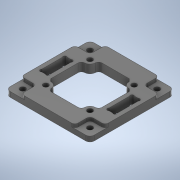
# Autodesk Inventor part: Camera_root_frame_e-CAM50_CUNX
Saved by Autodesk Inventor 2020.4 (Build 244396000, 396)
## iProperties
Part Number: Camera_root_frame_e-CAM50_CUNX
Material: アセタール樹脂、黒
Document SubType Name: Modeling
Designer: Masato Kubotera
Density: 1.425 g/cm^3
Appearance: 滑らか - 黒
Description: POM T5
Mass: 8.58066 g
Surface Area: 62.5532 cm^2
Volume: 6.02152 cm^3
Author: Masato Kubotera
Autodesk Inventor part; units mm, degrees
ref_plane "YZ Plane" through (0, 0, 0) normal (1, 0, 0) x (0, 1, 0)
ref_plane "XZ Plane" through (0, 0, 0) normal (0, 1, 0) x (-1, 0, 0)
ref_plane "XY Plane" through (0, 0, 0) normal (0, 0, 1) x (1, 0, 0)
derived "e-CAM50_CUNX.ipt"
sketch "スケッチ2" plane through (0, 0, 0) normal (0, 0, 1) x (1, 0, 0)
  line L0 (-22.5, 25) -> (22.5, 25)
  line L1 (25, 22.5) -> (25, -22.5)
  line L2 (22.5, -25) -> (-22.5, -25)
  line L3 (-25, -22.5) -> (-25, 22.5)
  line L4 (-25, 25) -> (25, -25) construction
  line L5 (25, 25) -> (-25, -25) construction
  arc A0 (-22.5, 25) -> (-25, 22.5) centre (-22.5, 22.5) ccw
  arc A1 (-25, -22.5) -> (-22.5, -25) centre (-22.5, -22.5) ccw
  arc A2 (22.5, -25) -> (25, -22.5) centre (22.5, -22.5) ccw
  arc A3 (25, 22.5) -> (22.5, 25) centre (22.5, 22.5) ccw
  line L6 (-25, -22.5) -> (25, -22.5) construction
  line L7 (25, -22.5) -> (25, -17.5)
  line L8 (25, -17.5) -> (-25, -17.5) construction
  line L9 (-25, -17.5) -> (-25, -22.5) construction
  line L10 (-25, -22.5) -> (25, -17.5) construction
  line L11 (25, -22.5) -> (-25, -17.5) construction
  line L12 (-25, -20) -> (25, -20) construction
  line L13 (0, 15) -> (0, -15) construction
  circle A4 centre (-20, -20) radius 1.6
  circle A5 centre (20, -20) radius 1.6
  line L14 (-15, 0) -> (15, 0) construction
  circle A6 centre (-20, 20) radius 1.6
  circle A7 centre (20, 20) radius 1.6
  circle A8 centre (-5.5, -9) radius 2 construction
  circle A9 centre (13.14, 13.14) radius 1.1 projected
  circle A10 centre (13.14, -13.14) radius 1.1 projected
  circle A11 centre (-13.14, -13.14) radius 1.1 projected
  circle A12 centre (-13.14, 13.14) radius 1.1 projected
  circle A13 centre (-13.14, -13.14) radius 1.55
  circle A14 centre (13.14, -13.14) radius 1.55
  circle A15 centre (13.14, 13.14) radius 1.55
  circle A16 centre (-13.14, 13.14) radius 1.55
  line L15 (-15, -15) -> (15, -15) projected
  line L16 (-15, 15) -> (-15, -15) projected
  line L17 (-15, -7.8919) -> (-15, 0)
  line L18 (0, -15) -> (-7.8919, -15)
  arc A17 (-9.8912, -13.0533) -> (-13.0533, -9.8912) centre (-13.14, -13.14) ccw
  arc A18 (-9.8912, -13.0533) -> (-7.8919, -15) centre (-7.8919, -13) ccw
  arc A19 (-15, -7.8919) -> (-13.0533, -9.8912) centre (-13, -7.8919) ccw
  line L19 (-15, 7.8919) -> (-15, 0)
  line L20 (0, 15) -> (-7.8919, 15)
  arc A20 (-13.0533, 9.8912) -> (-9.8912, 13.0533) centre (-13.14, 13.14) ccw
  arc A21 (-7.8919, 15) -> (-9.8912, 13.0533) centre (-7.8919, 13) ccw
  arc A22 (-13.0533, 9.8912) -> (-15, 7.8919) centre (-13, 7.8919) ccw
  line L21 (15, -7.8919) -> (15, 0)
  line L22 (0, -15) -> (7.8919, -15)
  arc A23 (13.0533, -9.8912) -> (9.8912, -13.0533) centre (13.14, -13.14) ccw
  arc A24 (7.8919, -15) -> (9.8912, -13.0533) centre (7.8919, -13) ccw
  arc A25 (13.0533, -9.8912) -> (15, -7.8919) centre (13, -7.8919) ccw
  arc A26 (15, 7.8919) -> (13.0533, 9.8912) centre (13, 7.8919) ccw
  arc A27 (9.8912, 13.0533) -> (7.8919, 15) centre (7.8919, 13) ccw
  line L23 (15, 7.8919) -> (15, 0)
  line L24 (0, 15) -> (7.8919, 15)
  arc A28 (9.8912, 13.0533) -> (13.0533, 9.8912) centre (13.14, 13.14) ccw
  line L25 (-7.5, -22.5) -> (7.5, -22.5) construction
  line L26 (7.5, -22.5) -> (7.5, -17.5) construction
  line L27 (7.5, -17.5) -> (-7.5, -17.5) construction
  line L28 (-7.5, -17.5) -> (-7.5, -22.5) construction
  line L29 (-7.5, -22.5) -> (7.5, -17.5) construction
  line L30 (7.5, -22.5) -> (-7.5, -17.5) construction
  line L31 (-6.0651, -22.55) -> (6.0651, -22.55)
  line L32 (6.0651, -17.45) -> (-6.0651, -17.45)
  arc A29 (-7.55, -21.0651) -> (-6.0651, -22.55) centre (-6.8075, -21.8075) ccw
  arc A30 (-6.0651, -17.45) -> (-7.55, -18.9349) centre (-6.8075, -18.1925) ccw
  arc A31 (6.0651, -22.55) -> (7.55, -21.0651) centre (6.8075, -21.8075) ccw
  arc A32 (7.55, -18.9349) -> (6.0651, -17.45) centre (6.8075, -18.1925) ccw
  line L33 (-7.55, -22.5) -> (-7.55, -22.55)
  line L34 (-7.55, -18.9349) -> (-7.55, -21.0651)
  line L35 (7.55, -21.0651) -> (7.55, -18.9349)
  line L36 (-6.0651, 22.55) -> (6.0651, 22.55)
  line L37 (6.0651, 17.45) -> (-6.0651, 17.45)
  arc A33 (-6.0651, 22.55) -> (-7.55, 21.0651) centre (-6.8075, 21.8075) ccw
  arc A34 (-7.55, 18.9349) -> (-6.0651, 17.45) centre (-6.8075, 18.1925) ccw
  arc A35 (6.0651, 17.45) -> (7.55, 18.9349) centre (6.8075, 18.1925) ccw
  arc A36 (7.55, 21.0651) -> (6.0651, 22.55) centre (6.8075, 21.8075) ccw
  line L38 (-7.55, 18.9349) -> (-7.55, 21.0651)
  line L39 (7.55, 21.0651) -> (7.55, 18.9349)
  arc A37 (-16, -18) -> (-18, -16) centre (-18, -18) ccw
  line L40 (-16, -18) -> (-16, -23)
  arc A38 (-15.9998, -22.9729) -> (-14, -25) centre (-14, -23) ccw
  line L41 (-16, 18) -> (-16, 23)
  arc A39 (-14, 25) -> (-15.9998, 22.9729) centre (-14, 23) ccw
  line L42 (16, -18) -> (16, -23)
  arc A40 (14, -25) -> (15.9998, -22.9729) centre (14, -23) ccw
  line L43 (16, 18) -> (16, 23)
  arc A41 (15.9998, 22.9729) -> (14, 25) centre (14, 23) ccw
  line L44 (15, 0) -> (-15, 0) construction
  arc A42 (-25, -14) -> (-23, -16) centre (-23, -14) ccw
  line L45 (-23, -16) -> (-18, -16)
  arc A43 (-18, 16) -> (-16, 18) centre (-18, 18) ccw
  arc A44 (-23, 16) -> (-25, 14) centre (-23, 14) ccw
  line L46 (-23, 16) -> (-18, 16)
  arc A45 (18, -16) -> (16, -18) centre (18, -18) ccw
  arc A46 (23, -16) -> (25, -14) centre (23, -14) ccw
  line L47 (23, -16) -> (18, -16)
  arc A47 (25, 14) -> (23, 16) centre (23, 14) ccw
  line L48 (23, 16) -> (18, 16)
  arc A48 (16, 18) -> (18, 16) centre (18, 18) ccw
  point P0 (0, 0)
  point P1 (0, -20)
  point P2 (0, -20)
  point P3 (-10.4749, -15)
  point P4 (-15, 7.8919)
  point P5 (7.8919, -15)
  point P6 (-7.8919, -15)
  point P7 (-16.5858, -16.5858)
  point P8 (14, -25)
  point P9 (14, 25)
  point P10 (-14, 25)
  point P11 (-25, 14)
  point P12 (25, 14)
  point P13 (-7.5968, -22.5)
  point P14 (7.5968, -22.5)
  point P15 (7.5968, 22.5)
  point P16 (-7.5968, 22.5)
  dimension "d1" = 50
  dimension "d2" = 50
  dimension "d3" = 2.5
  dimension "d7" = 5
  dimension "d8" = 5
  dimension "d9" = 3.2
  dimension "d10" = 5
  dimension "d12" = 3.1
  dimension "d20" = 2
  dimension "d21" = 40
  dimension "d23" = 12.5
  dimension "d24" = 15
  dimension "d27" = 0.05
  dimension "d28" = 1.05
  dimension "d30" = 0.05
  dimension "d33" = 10
  dimension "d39" = 2
  dimension "d40" = 2
  dimension "d41" = 4
  dimension "d46" = 15
  dimension "d59" = 4
  dimension "d60" = 2
  dimension "d61" = 3.25
  constraints: 90 end point, 79 point on circle, 77 symmetric about line, 44 centre point, 21 point on line, 18 tangent, 10 parallel, 9 midpoint, 5 coincident, 4 equal radius, 4 horizontal, 4 perpendicular, 2 collinear, 1 vertical, 31 other
  measures "d1" distance of L4.end L5.end
  measures "d2" distance of L5.start L4.end
  measures "d3" radius of A0
  measures "d7" distance of L7.end L6.end
  measures "d8" distance from line of L5.end L12
  measures "d9" diameter of A4
  measures "d10" distance of L12.start A4.centre
  measures "d12" diameter of A13
  measures "d20" radius of A18
  measures "d21" distance of A6.centre A4.centre
  measures "d23" horizontal distance of L25.start A4.centre
  measures "d24" distance of L25.end L25.start
  measures "d27" distance between parallel lines of L31 L25
  measures "d28" radius of A29
  measures "d30" distance between parallel lines of L28 L34
  measures "d33" distance from line of L1 L14.end
  measures "d39" radius of A38
  measures "d40" radius of A37
  measures "d41" horizontal distance of L40.end A4.centre
  measures "d46" distance of point (0, 0) L14.start
  measures "d59" distance from line of A4.centre L45
  measures "d60" radius of A42
  measures "d61" radius of A17
extrude "押し出し1" add sketch "スケッチ2" along normal blind 5 contours L0 A41 L43 A48 L48 A47 L1 A46 L47 A45 L42 A40 L2 A38 L40 A37 L45 A42 L3 A44 L46 A43 L41 A39 | L16 A19 A17 A18 L15
extrude "押し出し2" add sketch "スケッチ2" along normal blind 3 contours L0 A39 L41 A43 L46 A44 L3 A0 | L0 A3 L1 A47 L48 A48 L43 A41 | A42 L45 A37 L40 A38 L2 A1 L3 | L1 A2 L2 A40 L42 A45 L47 A46
sketch "スケッチ1" plane through (0, 0, 0) normal (0, 0, 1) x (1, 0, 0)
  line L0 (15, 15) -> (-15, 15) construction
  line L1 (-15, 15) -> (-15, -15) construction
  line L2 (-15, -15) -> (15, -15) construction
  line L3 (15, -15) -> (15, 15) construction
  line L4 (15, 15) -> (-15, -15) construction
  line L5 (-15, 15) -> (15, -15) construction
  line L6 (-13.14, 13.14) -> (13.14, 13.14) construction
  line L7 (13.14, 13.14) -> (13.14, -13.14) construction
  line L8 (13.14, -13.14) -> (-13.14, -13.14) construction
  line L9 (-13.14, -13.14) -> (-13.14, 13.14) construction
  line L10 (-13.14, 13.14) -> (13.14, -13.14) construction
  line L11 (13.14, 13.14) -> (-13.14, -13.14) construction
  circle A0 centre (-13.14, -13.14) radius 1.1 construction
  line L12 (-15, 0) -> (15, 0) construction
  line L13 (0, 15) -> (0, -15) construction
  circle A1 centre (-13.14, 13.14) radius 1.1 construction
  circle A2 centre (13.14, 13.14) radius 1.1 construction
  circle A3 centre (13.14, -13.14) radius 1.1 construction
  circle A4 centre (-13.14, -13.14) radius 2 construction
  circle A5 centre (-13.14, 13.14) radius 2 construction
  circle A6 centre (13.14, -13.14) radius 2 construction
  circle A7 centre (13.14, 13.14) radius 2 construction
  circle A8 centre (0, 0) radius 7 construction
  circle A9 centre (-5.5, -9) radius 2 construction
  line L14 (-7, 8) -> (7, 8) projected
  line L15 (8, 7) -> (8, -7) projected
  line L16 (7, -8) -> (-7, -8) projected
  line L17 (-8, -7) -> (-8, 7) projected
  line L18 (-8, 8) -> (8, -8) construction
  line L19 (8, 8) -> (-8, -8) construction
  arc A10 (-7, 8) -> (-8, 7) centre (-7, 7) ccw projected
  arc A11 (-8, -7) -> (-7, -8) centre (-7, -7) ccw projected
  arc A12 (7, -8) -> (8, -7) centre (7, -7) ccw projected
  arc A13 (8, 7) -> (7, 8) centre (7, 7) ccw projected
  arc A14 (-10, 2) -> (-10, -2) centre (-10, 0) ccw projected
  line L20 (-10, 2) -> (-8, 2) projected
  line L21 (-10, -2) -> (-8, -2) projected
  line L22 (10, 2) -> (8, 2) projected
  arc A15 (10, -2) -> (10, 2) centre (10, 0) ccw projected
  line L23 (10, -2) -> (8, -2) projected
  constraints: 1 centre point
equation "\"d27\" = d26"
equation "\"d40\" = d39"
equation "\"d26\" = 0.05"
